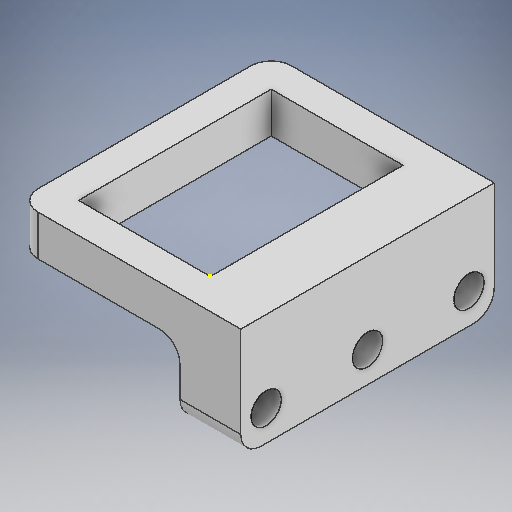
# Autodesk Inventor part: power_button_holder
Saved by Autodesk Inventor 2026.1 (Build 301233000, 233)
## iProperties
Created: 2025-12-03
Part Number: power_button_holder
Material: Generic
Document SubType Name: Modeling
Designer: emanuel
Density: 1 g/cm^3
Appearance: Default
Author: emanuel
Autodesk Inventor part; units mm, degrees
ref_plane "YZ Plane" through (0, 0, 0) normal (1, 0, 0) x (0, 1, 0)
ref_plane "XZ Plane" through (0, 0, 0) normal (0, 1, 0) x (-1, 0, 0)
ref_plane "XY Plane" through (0, 0, 0) normal (0, 0, 1) x (1, 0, 0)
sketch "Sketch1" plane through (0, 0, 0) normal (0, 1, 0) x (-1, 0, 0)
  line L0 (0, 0) -> (13, 0)
  line L1 (13, 0) -> (13, -19)
  line L2 (13, -19) -> (0, -19)
  line L3 (0, -19) -> (0, 0)
  line L4 (0, 0) -> (-3, 0)
  line L5 (-3, 0) -> (-3, 3)
  line L6 (-3, 3) -> (0, 3)
  line L7 (0, 3) -> (0, 0)
  line L8 (13, -19) -> (16, -19)
  line L9 (16, -19) -> (16, -22)
  line L10 (16, -22) -> (13, -22)
  line L11 (13, -22) -> (13, -19)
  line L12 (16, -22) -> (-3, -22)
  line L13 (-3, -22) -> (-3, 3)
  line L14 (-3, 3) -> (16, 3)
  line L15 (16, 3) -> (16, -22)
  dimension "d0" = 13
  dimension "d1" = 19
  dimension "d2" = 3
  dimension "d3" = 3
  dimension "d4" = 3
  dimension "d5" = 3
  constraints: 32 end point, 8 parallel, 4 horizontal, 4 perpendicular
  measures "d0" distance of L1.end L2.end
  measures "d1" distance of L0.end L1.end
  measures "d2" distance of L5.end L6.end
  measures "d3" distance of L4.end L5.end
  measures "d4" distance of L9.end L10.end
  measures "d5" distance of L8.end L9.end
extrude "Extrusion1" add sketch "Sketch1" along normal blind 4 contours L7 L14 L15 L8 L1 L0 | L3 L2 L11 L12 L13 L4 | L4 L5 L6 L7 | L8 L9 L10 L11
sketch "Sketch2" plane through (3, 0, 3) normal (1, 0, 0) x (0, 0, -1)
  line L0 (25, 0) -> (25, 4) projected
  line L1 (25, 0) -> (0, 0) projected
  line L2 (25, 0) -> (0, 0)
  line L3 (25, 0) -> (12.5, 0)
  line L4 (3, 0) -> (22, 0) projected
  line L5 (12.5, 0) -> (12.5, -4)
  circle A0 centre (12.5, -4) radius 1.5
  line L6 (12.5, -4) -> (22.5, -4)
  line L7 (22.5, -4) -> (2.5, -4)
  circle A1 centre (2.5, -4) radius 1.5
  circle A2 centre (22.5, -4) radius 1.5
  line L8 (0, 0) -> (25, 0)
  line L9 (25, 0) -> (25, -7)
  line L10 (25, -7) -> (0, -7)
  line L11 (0, -7) -> (0, 0)
  line L12 (25, 0) -> (25, 4) projected
  line L13 (0, 0) -> (25, 0)
  line L14 (25, 0) -> (25, 4)
  line L15 (25, 4) -> (0, 4)
  line L16 (0, 4) -> (0, 0)
  dimension "d8" = 12.5
  dimension "d9" = 4
  dimension "d10" = 3
  dimension "d11" = 10
  dimension "d12" = 20
  dimension "d13" = 3
  dimension "d14" = 3
  dimension "d15" = 7
  constraints: 26 end point, 4 horizontal, 4 parallel, 3 centre point, 3 coincident, 3 perpendicular, 1 midpoint, 1 point on line
  measures "d8" distance of L0.start L3.end
  measures "d9" distance of L3.end L5.end
  measures "d10" diameter of A0
  measures "d11" distance of L6.start L6.end
  measures "d12" distance of L6.end L7.end
  measures "d13" diameter of A1
  measures "d14" diameter of A2
  measures "d15" distance of L8.end L9.end
extrude "Extrusion2" add sketch "Sketch2" along normal mid plane 6
fillet "Fillet1" radius 2 4 edges at (-16, 2, -22) (-16, 2, 3) (3, -7, 3) (3, -7, -22)
fillet "Fillet2" radius 2 2 edges at (0, 0, -20.5) (0, 0, 1.5)
sketch "Sketch3" plane through (0, 4, 0) normal (0, 1, 0) x (1, 0, 0)
  point P0 (0, 0)
body "Solid1"
